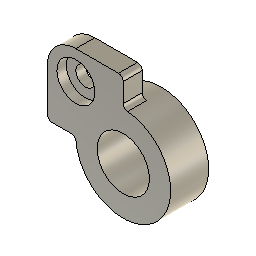
lesson 8 improving with sketch (Autodesk Fusion 360 design; units mm, degrees)
part number: 2025-09-12-21-03-01-169
Autodesk Fusion 360 part; units mm, degrees
sketch "Sketch1" plane through (0, 0, 0) normal (0, 1, 0) x (1, 0, 0)
  circle A0 centre (0, 0) radius 17.4625
  circle A1 centre (0, 0) radius 31.75
  line L0 (-50.8, -50.8) -> (0, -50.8)
  line L1 (0, -50.8) -> (0, 0)
  line L2 (0, 0) -> (-50.8, 0)
  line L3 (-50.8, 0) -> (-50.8, -50.8)
  circle A2 centre (-31.75, -31.75) radius 1.27
  dimension "d1" = 34.925
  dimension "d2" = 63.5
  dimension "d3" = 50.8
  dimension "d4" = 50.8
  dimension "d5" = 31.75
  dimension "d6" = 31.75
  dimension "d7" = 2.54
  constraint coincident A0.centre A1.centre
  constraint horizontal L0
  constraint vertical L1
  constraint horizontal L2
  constraint vertical L3
  measures "d1" diameter of A0
  measures "d2" diameter of A1
  measures "d3" distance of L0.start L0.end
  measures "d4" distance of L0.start L2.end
  measures "d5" distance of L1 A2.centre
  measures "d6" distance of L2 A2.centre
  measures "d7" diameter of A2
extrude "Extrude1" add sketch "Sketch1" along normal blind 25.4 contours A0 A1 L1 L2 | A0 A1 L1 L2
extrude "Extrude2" add sketch "Sketch1" along normal blind 12.7 contours A1 L0 L1 L2 L3
fillet "Fillet1" radius 19.05 1 edges at (-50.8, 6.35, 50.8)
fillet "Fillet1" radius 3.175 4 edges at (0, 6.35, 50.8) (0, 6.35, 31.75) (-50.8, 6.35, 0) (-31.75, 6.35, 0)
hole "Hole1" at (-31.75, 0, 31.75) direction (0, 1, 0) diameter 12.7 depth 25.4 tip angle 118 counterbore diameter 25.4 counterbore depth 6.35
equation "d2 = ( 1.25 * 2 ) * 1 in"
